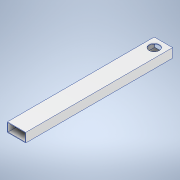
# Autodesk Inventor part: 2x1 Support
Saved by Autodesk Inventor 2020 (Build 240168000, 168)
## iProperties
Created: 2020-01-13
Part Number: 2x1 Support
Material: Aluminum 6061
Document SubType Name: Modeling
Designer: autum
Density: 2.7 g/cm^3
Appearance: Aluminum - Flat
Author: autum
Autodesk Inventor part; units mm, degrees
ref_plane "YZ Plane" through (0, 0, 0) normal (1, 0, 0) x (0, 1, 0)
ref_plane "XZ Plane" through (0, 0, 0) normal (0, 1, 0) x (-1, 0, 0)
ref_plane "XY Plane" through (0, 0, 0) normal (0, 0, 1) x (1, 0, 0)
sketch "Sketch1" plane through (0, 0, 0) normal (0, 0, 1) x (1, 0, 0)
  line L0 (-25.4, -12.7) -> (25.4, -12.7)
  line L1 (25.4, -12.7) -> (25.4, 12.7)
  line L2 (25.4, 12.7) -> (-25.4, 12.7)
  line L3 (-25.4, 12.7) -> (-25.4, -12.7)
  line L4 (-25.4, -12.7) -> (25.4, 12.7) construction
  line L5 (25.4, -12.7) -> (-25.4, 12.7) construction
  line L6 (-23.8125, -11.1125) -> (23.8125, -11.1125)
  line L7 (23.8125, -11.1125) -> (23.8125, 11.1125)
  line L8 (23.8125, 11.1125) -> (-23.8125, 11.1125)
  line L9 (-23.8125, 11.1125) -> (-23.8125, -11.1125)
  line L10 (-23.8125, -11.1125) -> (23.8125, 11.1125) construction
  line L11 (23.8125, -11.1125) -> (-23.8125, 11.1125) construction
  point P0 (0, 0)
  dimension "d0" = 50.8
  dimension "d1" = 25.4
  dimension "d2" = 47.625
  dimension "d3" = 22.225
  constraints: 24 end point, 4 midpoint, 4 parallel, 2 horizontal, 2 perpendicular
  measures "d0" distance of L2.end L1.end
  measures "d1" distance of L1.end L0.end
  measures "d2" distance of L8.end L7.end
  measures "d3" distance of L7.end L6.end
extrude "Extrusion1" add sketch "Sketch1" along normal blind 406.4
sketch "Sketch2" plane through (-25.4, 12.7, 0) normal (0, 1, 0) x (1, 0, 0)
  line L0 (0, 0) -> (0, -406.4) projected
  point P0 (25.4, 0)
  point P1 (25.4, -25.4)
  dimension "d13" = 25.4
  dimension "d14" = 25.4
  measures "d13" distance of point (25.4, 0) point (25.4, -25.4)
  measures "d14" distance from line of L0 point (25.4, -25.4)
hole "Hole1" at (0, 12.7, 25.4) direction (0, -1, 0) diameter 28.575 end through all
body "Solid1"
